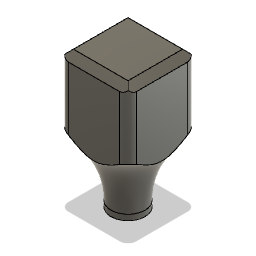
fillet_chamfer_exercise (Autodesk Fusion 360 design; units mm, degrees)
Autodesk Fusion 360 part; units mm, degrees
sketch "Sketch1" plane through (0, 0, 0) normal (0, 0, 1) x (1, 0, 0)
  line L0 (10, -10) -> (-10, -10)
  line L1 (-10, -10) -> (-10, 10)
  line L2 (-10, 10) -> (10, 10)
  line L3 (10, 10) -> (10, -10)
  line L4 (10, -10) -> (-10, 10) construction
  line L5 (-10, -10) -> (10, 10) construction
  dimension "d1" = 20
  dimension "d2" = 20
  constraint horizontal L0
  constraint perpendicular L0 L1
  constraint parallel L0 L2
  constraint parallel L1 L3
  constraint coincident L4 origin
  constraint coincident L5 origin
  measures "d1" distance of L1.end L2.end
  measures "d2" distance of L0.end L1.end
extrude "Extrude1" add sketch "Sketch1" along normal mid plane 20
sketch "Sketch2" plane through (0, -10, 0) normal (0, -1, 0) x (1, 0, 0)
  line L0 (10, -10) -> (10, 10)
  line L1 (10, 10) -> (-10, 10)
  line L2 (-10, 10) -> (-10, -10)
  line L3 (-10, -10) -> (10, -10)
  circle A0 centre (0, 0) radius 5
  dimension "d5" = 10
  constraint coincident A0.centre origin
  measures "d5" diameter of A0
extrude "Extrude2" add sketch "Sketch2" along normal blind 20 contours A0
chamfer "Chamfer1" distance 2 angle 45 4 edges at (-10, 10, 0) (0, 10, -10) (10, 10, 0) (0, 10, 10)
fillet "Fillet2" radius 2.5 4 edges at (-10, -1, 10) (-10, -1, -10) (10, -1, 10) (10, -1, -10)
chamfer "Chamfer2" distance 8 angle 45 1 edges at (-4.6616, -10, 1.8081)
fillet "Fillet1" radius 25 1 edges at (-4.6616, -18, 1.8081)
